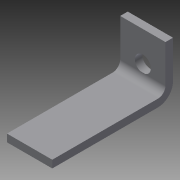
# Autodesk Inventor part: pawl mount reinforcement
Saved by Autodesk Inventor 2013 (Build 170138000, 138)
## iProperties
Created: 2013-02-05
Part Number: pawl mount reinforcement
Material: Generic
Document SubType Name: Sheet Metal
Designer: Arpan
Density: 1 g/cm^3
Sheet Metal Rule: Default
Author: Arpan
Autodesk Inventor part; units mm, degrees
ref_plane "YZ Plane" through (0, 0, 0) normal (1, 0, 0) x (0, 1, 0)
ref_plane "XZ Plane" through (0, 0, 0) normal (0, 1, 0) x (-1, 0, 0)
ref_plane "XY Plane" through (0, 0, 0) normal (0, 0, 1) x (1, 0, 0)
sketch "Sketch1" plane through (0, 0, 0) normal (0, 0, 1) x (1, 0, 0)
  line L0 (0, 0) -> (0, -22.225)
  line L1 (0, 0) -> (-19.05, 0)
  line L2 (-19.05, 0) -> (-19.05, -22.225)
  line L3 (-19.05, -22.225) -> (0, -22.225)
  dimension "d0" = 22.225
  dimension "d1" = 19.05
  measures "d0" distance of L0.start L0.end
  measures "d1" distance of L0.start L1.end
extrude "Plate1" add sketch "Sketch1" along normal blind 3.175
sketch "Sketch2" plane through (0, -19.05, 0) normal (0, -1, 0) x (1, 0, 0)
  line L0 (-19.05, 0) -> (0, 0)
  line L1 (0, 0) -> (0, 76.2)
  line L2 (0, 76.2) -> (-19.05, 76.2)
  line L3 (-19.05, 76.2) -> (-19.05, 0)
  constraints: 6 end point, 1 horizontal, 1 perpendicular, 1 vertical
edge flange "Flange1" height 76.2 angle 90 thickness 3.175 bend radius 1.27 thickness toward (0, -1, 0) relief tear relief width 3.175 relief depth 1.5875 edges at (-9.525, -22.225, 3.175) wall of the first edge with corners at (-19.05, -19.05, 0) (0, -19.05, 0) (0, -19.05, 76.2) (-19.05, -19.05, 76.2)
bend "Bend1"
corner "Corner1"
sketch "Sketch3" plane through (0, 0, 3.175) normal (0, 0, 1) x (1, 0, 0)
  circle A0 centre (90.7515, -113.3098) radius 3.3782 projected
  circle A1 centre (90.7515, -113.3098) radius 3.3782 projected
  circle A2 centre (-9.525, -12.7) radius 3.3782 projected
extrude "Cut1" cut sketch "Sketch3" against normal blind 3.175 contours A2
sketch "Sketch4" plane through (-19.05, -19.05, 76.2) normal (0, 1, 0) x (1, 0, 0)
  line L0 (0, 0) -> (19.05, 0) projected
  line L1 (19.05, 0) -> (19.05, 71.755) projected
  line L2 (9.525, 0) -> (9.525, 12.7)
  circle A0 centre (9.525, 12.7) radius 3.3782
  line L3 (9.525, 12.7) -> (9.525, 25.4)
  circle A1 centre (9.525, 25.4) radius 3.3782
  point P0 (19.05, 76.2)
  dimension "d15" = 12.7
  dimension "d16" = 6.7564
  dimension "d17" = 12.7
  dimension "d18" = 6.7564
  constraints: 4 end point, 2 centre point, 2 coincident, 1 collinear, 1 midpoint, 1 parallel
  measures "d15" distance of L2.start L2.end
  measures "d16" diameter of A0
  measures "d17" distance of L3.start L3.end
  measures "d18" diameter of A1
extrude "Cut2" cut sketch "Sketch4" against normal blind 3.175
equation "\"d13\" = Thickness"
equation "\"d19\" = Thickness"
equation "\"d3\" = BendReliefWidth"
equation "\"d4\" = BendReliefDepth"
equation "\"d5\" = MinimumRemnant"
equation "\"d6\" = BendRadius"
equation "\"d10\" = CornerReliefSize"
equation "\"d11\" = GapSize"
equation "\"d12\" = JacobiRadiusSize"
equation "\"BendRadius\" = Thickness"
equation "\"BendReliefWidth\" = Thickness"
equation "\"BendReliefDepth\" = 0.5 * Thickness"
equation "\"CornerReliefSize\" = 4 * Thickness"
equation "\"MinimumRemnant\" = 2 * Thickness"
equation "\"TransitionRadius\" = BendRadius"
equation "\"JacobiRadiusSize\" = Thickness"
equation "\"GapSize\" = Thickness"
equation "\"d2\" = BendRadius"
equation "\"Thickness\" = 3.175"
body "Solid1"
